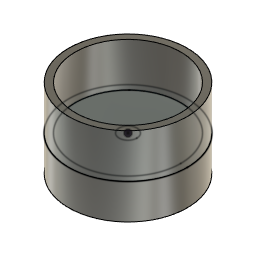
Aquazepp_LagerSchlagwerkzeug v3 (Autodesk Fusion 360 design; units mm, degrees)
Autodesk Fusion 360 part; units mm, degrees
sketch "Skizze1" plane through (0, 0, 0) normal (0, 0, 1) x (1, 0, 0)
  circle A0 centre (0, 0) radius 13.5
  circle A1 centre (0, 0) radius 12
  circle A2 centre (0, 0) radius 2
  dimension "d1" = 27
  dimension "d2" = 24
  dimension "d3" = 4
  constraint coincident A0.centre A1.centre
  constraint concentric A0 A1
  constraint concentric A1 A2
  measures "d1" diameter of A0
  measures "d2" diameter of A1
  measures "d3" diameter of A2
extrude "Extrusion1" add sketch "Skizze1" along normal blind 10 contours A0
extrude "Extrusion2" add sketch "Skizze1" against normal blind 8 contours A0 | A1
sketch "Skizze2" plane through (0, 0, -8) normal (0, 0, -1) x (1, 0, 0)
  circle A0 centre (0, 0) radius 2
  circle A1 centre (0, 0) radius 13.5
  circle A2 centre (0, 0) radius 13.5
  circle A3 centre (0, 0) radius 11.5
  dimension "d8" = -2
extrude "Extrusion3" cut sketch "Skizze2" against normal blind 2 contours A3
named bodies: "Aquazepp_LagerSchlagwerkzeug"
